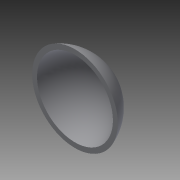
# Autodesk Inventor part: Spare part
Saved by Autodesk Inventor 2013 (Build 170138000, 138)
## iProperties
Created: 2014-07-07
Part Number: Spare part
Material: Genérico
Document SubType Name: Chapa
Designer: Administrador
Density: 1 g/cm^3
Sheet Metal Rule: Por defecto_mm
Author: Administrador
Autodesk Inventor part; units mm, degrees
ref_plane "YZ Plane" through (0, 0, 0) normal (1, 0, 0) x (0, 1, 0)
ref_plane "XZ Plane" through (0, 0, 0) normal (0, 1, 0) x (-1, 0, 0)
ref_plane "XY Plane" through (0, 0, 0) normal (0, 0, 1) x (1, 0, 0)
sketch "Boceto1" plane through (0, 0, 0) normal (0, 0, 1) x (1, 0, 0)
  arc A0 (18.8027, 6.816) -> (-0.0144, 20) centre (0, 0) ccw
  arc A1 (16.6596, 6.816) -> (-0.0122, 18) centre (0, 0) ccw
  line L0 (0, 0) -> (16.65, 0) construction
  line L1 (16.65, 6.816) -> (16.65, 6.8394) construction
  line L2 (-0.0122, 18) -> (-0.0144, 20)
  line L3 (-0.032, 6.816) -> (0, 6.816)
  line L4 (16.65, 6.816) -> (18.8027, 6.816)
  dimension "d2" = 40
  dimension "d3" = 36
  dimension "d4" = 16.65
  constraints: 10 end point, 5 point on circle, 2 centre point, 1 point on line
  measures "d2" diameter of A0
  measures "d3" diameter of A1
  measures "d4" distance of L0.start L0.end
revolve "Revolución1" add sketch "Boceto1" angle 360 about axis through (-0.0122, 18, 0) along (-0.0011, 1, 0)
equation "\"Radio_pliegue\" = Grosor"
equation "\"Anchura_desahogo_plegado\" = Grosor"
equation "\"Profundidad_desahogo_plegado\" = 0.5 * Grosor"
equation "\"Tamaño_destalonado\" = 4 * Grosor"
equation "\"Remanente_mínimo\" = 2 * Grosor"
equation "\"Radiodetransición\" = Radio_pliegue"
equation "\"Tamaño_de_radio_de_Jacobi\" = Radio_pliegue"
equation "\"TamañoSeparación\" = Grosor"
equation "\"Grosor\" = 0.5"
